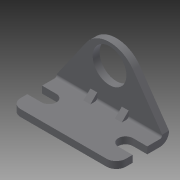
# Autodesk Inventor part: D-770
Saved by Autodesk Inventor 2013 (Build 170138000, 138)
## iProperties
Category: PARTsolutions
Company: BIMBA
Created: 2013-01-26
Part Number: D-770
Material: Generic
Catalog Web Link: www.cadenas.de
Description: Mounting Brackets for Original Line Cylinders-
Vendor: BIMBA
Document SubType Name: Modeling
Designer: actoennies
Manufacturer: BIMBA
Density: 1 g/cm^3
Mass: 1.92593 g
Surface Area: 20.9427 cm^2
Volume: 1.92593 cm^3
PSOL_IDENT_0: {\\10.0.0.242\data_v9\23d-libs\bimba\bimba\bimba_imperial\bimba_full_line\original_line_cylinders\ac
PSOL_IDENT_1: cessories\mounting_bracket.prj},191 {VTYP=3D},{NB=D-770},{LINA=D-770},{NN=Mounting Brackets for Orig
PSOL_IDENT_2: inal Line Cylinders},{DATE=26.09.2012 12:25:43},{GEOMDATE=27.08.2012 00:00:00},{VERSION=},{LINEID=40
PSOL_IDENT_3: },{LINESUBID=-1},{WBVAR=}  {NB=D-770},{LINA=D-770},{KT=DUMMY},{PN=D-770},{PSPN=0.44 (D-770)},{PN1=D-
PSOL_IDENT_4: 770},{MAT=Zinc-Plated Carbon Steel},{A=0.83},{A1=0.82900},{B=1.38},{B1=1.37500},{C=0.69},{C1=0.69000
PSOL_IDENT_5: },{D=0.44},{D1=0.44050},{E=0.19},{E1=0.19200},{F=0.38},{F1=0.38000},{G=0.56},{G1=0.56170},{H=0.09},{
PSOL_IDENT_6: H1=0.08970},{I=0.38},{I1=0.37500},{J=1.00},{J1=1.00000},{K=0.13},{K1=0.12500},{L=0.13},{L1=0.12500},
PSOL_IDENT_7: {M=0.03100},{N=0.00000},{SHP=3},{ASSCFGPRA=mounting_bracket3},{COLOR=0.75,0.75,0.75,0.00}
CNS_NB: D-770
CNS_NBSYN: $PN1.
CNS_LINA: D-770
CNS_PN: D-770
CNS_PSPN: ø.44 (D-770)
CNS_PN1: D-770
CNS_MAT: Zinc-Plated Carbon Steel
CNS_A: 0.83
CNS_A1: 0.82900
CNS_B: 1.38
CNS_B1: 1.37500
CNS_C: 0.69
CNS_C1: 0.69000
CNS_D: 0.44
CNS_D1: 0.44050
CNS_E: 0.19
CNS_E1: 0.19200
CNS_F: 0.38
CNS_F1: 0.38000
CNS_G: 0.56
CNS_G1: 0.56170
CNS_H: 0.09
CNS_H1: 0.08970
CNS_I: 0.38
CNS_I1: 0.37500
CNS_J: 1.00
CNS_J1: 1.00000
CNS_K: 0.13
CNS_K1: 0.12500
CNS_L: 0.13
CNS_L1: 0.12500
CNS_M: 0.03100
CNS_N: 0.00000
CNS_SHP: 3
CNS_ASSCFGPRA: mounting_bracket3
CNS_COLOR: 0.75,0.75,0.75,0.00
SUPPLIER: BIMBA
ARTICLENO: D-770
BOMINFO: D-770
CREATOR: CADENAS GmbH
Title: D-770
Author: Cadenas PARTsolutions
Autodesk Inventor part; units mm, degrees
sketch "Sketch_1" plane through (0, 0, 0) normal (1, 0, 0) x (0, 1, 0)
  line L0 (0, 17.526) -> (0, 3.0658)
  arc A0 (0, 3.0658) -> (3.0658, 0) centre (3.0658, 3.0658) ccw
  line L1 (3.0658, 0) -> (25.2679, 0)
  line L2 (25.2679, 0) -> (25.2679, 2.2784)
  line L3 (25.2679, 2.2784) -> (3.0658, 2.2784)
  arc A1 (2.2784, 3.0658) -> (3.0658, 2.2784) centre (3.0658, 3.0658) ccw
  line L4 (2.2784, 3.0658) -> (2.2784, 17.526)
  line L5 (2.2784, 17.526) -> (0, 17.526)
  constraints: 12 end point, 4 point on circle, 2 centre point
extrude "Extrusion1" add sketch "Sketch_1" along normal blind 34.925
sketch "Sketch_2" plane through (0, 0, 0) normal (0, 0, 1) x (1, 0, 0)
  line L0 (-6.985, -2.1057) -> (41.91, -2.1057)
  line L1 (41.91, -2.1057) -> (41.91, 33.6906)
  line L2 (41.91, 33.6906) -> (-6.985, 33.6906)
  line L3 (-6.985, 33.6906) -> (-6.985, -2.1057)
  line L4 (-2.2193, 0) -> (37.1443, 0)
  line L5 (37.1443, 0) -> (25.2694, 16.9886)
  arc A0 (25.2694, 16.9886) -> (9.6556, 16.9886) centre (17.4625, 11.5316) ccw
  line L6 (9.6556, 16.9886) -> (-2.2193, 0)
  constraints: 14 end point, 2 point on circle, 1 centre point
extrude "Extrusion2" cut sketch "Sketch_2" along normal blind 3.4176
sketch "Sketch3" plane through (34.925, 3.0658, 0) normal (0, 0, -1) x (-1, 0, 0)
  point P0 (17.4625, 11.2014)
hole "Drilling 1" at (17.4625, 14.2672, 0) direction (0, 0, 1) diameter 11.1887 depth 3.4176
sketch "Sketch_6" plane through (0, 0, 0) normal (0, 1, 0) x (-1, 0, 0)
  line L0 (17.4625, 14.351) -> (17.4625, 22.352)
  line L1 (17.4625, 22.352) -> (-3.175, 22.352)
  line L2 (-3.175, 22.352) -> (-3.175, 17.526)
  arc A0 (0, 14.351) -> (-3.175, 17.526) centre (-3.175, 14.351) ccw
  line L3 (0, 14.351) -> (17.4625, 14.351)
  constraints: 8 end point, 2 point on circle, 1 centre point
extrude "Extrusion3" cut sketch "Sketch_6" along normal blind 3.4176
sketch "Sketch_7" plane through (0, 0, 0) normal (0, 1, 0) x (-1, 0, 0)
  line L0 (-31.75, 22.352) -> (-52.3875, 22.352)
  line L1 (-52.3875, 22.352) -> (-52.3875, 14.351)
  line L2 (-52.3875, 14.351) -> (-34.925, 14.351)
  arc A0 (-31.75, 17.526) -> (-34.925, 14.351) centre (-31.75, 14.351) ccw
  line L3 (-31.75, 17.526) -> (-31.75, 22.352)
  constraints: 8 end point, 2 point on circle, 1 centre point
extrude "Extrusion4" cut sketch "Sketch_7" along normal blind 3.4176
sketch "Sketch_8" plane through (0, 0, 0) normal (0, 1, 0) x (-1, 0, 0)
  line L0 (3.4925, 12.0904) -> (-4.7625, 12.0904)
  arc A0 (-4.7625, 12.0904) -> (-4.7625, 7.2136) centre (-4.7625, 9.652) ccw
  line L1 (-4.7625, 7.2136) -> (3.4925, 7.2136)
  line L2 (3.4925, 7.2136) -> (3.4925, 12.0904)
  constraints: 6 end point, 2 point on circle, 1 centre point
extrude "Extrusion5" cut sketch "Sketch_8" along normal blind 3.4176
sketch "Sketch_9" plane through (0, 0, 0) normal (0, 1, 0) x (-1, 0, 0)
  arc A0 (-30.1625, 7.2136) -> (-30.1625, 12.0904) centre (-30.1625, 9.652) ccw
  line L0 (-30.1625, 12.0904) -> (-38.4175, 12.0904)
  line L1 (-38.4175, 12.0904) -> (-38.4175, 7.2136)
  line L2 (-38.4175, 7.2136) -> (-30.1625, 7.2136)
  constraints: 6 end point, 2 point on circle, 1 centre point
extrude "Extrusion6" cut sketch "Sketch_9" along normal blind 3.4176
sketch "Sketch_10" plane through (11.1125, 0, 0) normal (1, 0, 0) x (0, 0, -1)
  arc A0 (-4.5568, 1.8456) -> (-1.8456, 4.5568) centre (-3.0658, 3.0658) ccw
  line L0 (-1.8456, 4.5568) -> (-2.2784, 4.5568)
  line L1 (-2.2784, 4.5568) -> (-4.5568, 2.2784)
  line L2 (-4.5568, 2.2784) -> (-4.5568, 1.8456)
  constraints: 6 end point, 2 point on circle, 1 centre point
extrude "Extrusion7" add sketch "Sketch_10" along normal blind 2.2784
sketch "Sketch_14" plane through (23.8125, 0, 0) normal (1, 0, 0) x (0, 0, -1)
  arc A0 (-4.5568, 1.8456) -> (-1.8456, 4.5568) centre (-3.0658, 3.0658) ccw
  line L0 (-1.8456, 4.5568) -> (-2.2784, 4.5568)
  line L1 (-2.2784, 4.5568) -> (-4.5568, 2.2784)
  line L2 (-4.5568, 2.2784) -> (-4.5568, 1.8456)
  constraints: 6 end point, 2 point on circle, 1 centre point
extrude "Extrusion8" add sketch "Sketch_14" against normal blind 2.2784
ref_plane "h1_XY" through (17.4625, 0, 17.526) normal (1, 0, 0) x (0, 0, -1)
ref_plane "h1_YZ" through (17.4625, 0, 17.526) normal (0, 0, -1) x (0, 1, 0)
ref_plane "h1_ZX" through (17.4625, 0, 17.526) normal (0, 1, 0) x (1, 0, 0)
ref_plane "d1_XY" through (17.4625, 8.6728, 0) normal (1, 0, 0) x (0, 0, -1)
ref_plane "d1_YZ" through (17.4625, 8.6728, 0) normal (0, 0, -1) x (0, 1, 0)
ref_plane "d1_ZX" through (17.4625, 8.6728, 0) normal (0, 1, 0) x (1, 0, 0)
ref_plane "h2_XY" through (17.4625, 2.2784, 17.526) normal (1, 0, 0) x (0, 0, -1)
ref_plane "h2_YZ" through (17.4625, 2.2784, 17.526) normal (0, 0, -1) x (0, 1, 0)
ref_plane "h2_ZX" through (17.4625, 2.2784, 17.526) normal (0, 1, 0) x (1, 0, 0)
ref_plane "d2_XY" through (17.4625, 19.8615, 0) normal (1, 0, 0) x (0, 0, -1)
ref_plane "d2_YZ" through (17.4625, 19.8615, 0) normal (0, 0, -1) x (0, 1, 0)
ref_plane "d2_ZX" through (17.4625, 19.8615, 0) normal (0, 1, 0) x (1, 0, 0)
ref_plane "h3_XY" through (17.4625, 14.2672, 2.2784) normal (1, 0, 0) x (0, 0, -1)
ref_plane "h3_YZ" through (17.4625, 14.2672, 2.2784) normal (0, 0, -1) x (0, 1, 0)
ref_plane "h3_ZX" through (17.4625, 14.2672, 2.2784) normal (0, 1, 0) x (1, 0, 0)
ref_plane "h4_XY" through (17.4625, 21.0566, 2.2784) normal (1, 0, 0) x (0, 0, -1)
ref_plane "h4_YZ" through (17.4625, 21.0566, 2.2784) normal (0, 0, -1) x (0, 1, 0)
ref_plane "h4_ZX" through (17.4625, 21.0566, 2.2784) normal (0, 1, 0) x (1, 0, 0)
ref_plane "h5_XY" through (34.925, 3.175, 0) normal (1, 0, 0) x (0, 0, -1)
ref_plane "h5_YZ" through (34.925, 3.175, 0) normal (0, 0, -1) x (0, 1, 0)
ref_plane "h5_ZX" through (34.925, 3.175, 0) normal (0, 1, 0) x (1, 0, 0)
ref_plane "h6_XY" through (34.925, 0, 0) normal (1, 0, 0) x (0, 0, -1)
ref_plane "h6_YZ" through (34.925, 0, 0) normal (0, 0, -1) x (0, 1, 0)
ref_plane "h6_ZX" through (34.925, 0, 0) normal (0, 1, 0) x (1, 0, 0)
ref_plane "l1_XY" through (0, 0, 0) normal (0, 1, 0) x (1, 0, 0)
ref_plane "l1_YZ" through (0, 0, 0) normal (1, 0, 0) x (0, 0, -1)
ref_plane "l1_ZX" through (0, 0, 0) normal (0, 0, -1) x (0, 1, 0)
ref_plane "l2_XY" through (34.925, 0, 0) normal (0, 1, 0) x (1, 0, 0)
ref_plane "l2_YZ" through (34.925, 0, 0) normal (1, 0, 0) x (0, 0, -1)
ref_plane "l2_ZX" through (34.925, 0, 0) normal (0, 0, -1) x (0, 1, 0)
ref_plane "l3_XY" through (0, 0, 17.526) normal (0, 1, 0) x (1, 0, 0)
ref_plane "l3_YZ" through (0, 0, 17.526) normal (1, 0, 0) x (0, 0, -1)
ref_plane "l3_ZX" through (0, 0, 17.526) normal (0, 0, -1) x (0, 1, 0)
ref_plane "l4_XY" through (0, 0, 9.652) normal (0, 1, 0) x (1, 0, 0)
ref_plane "l4_YZ" through (0, 0, 9.652) normal (1, 0, 0) x (0, 0, -1)
ref_plane "l4_ZX" through (0, 0, 9.652) normal (0, 0, -1) x (0, 1, 0)
ref_plane "l5_XY" through (4.7625, 0, 9.652) normal (0, 1, 0) x (1, 0, 0)
ref_plane "l5_YZ" through (4.7625, 0, 9.652) normal (1, 0, 0) x (0, 0, -1)
ref_plane "l5_ZX" through (4.7625, 0, 9.652) normal (0, 0, -1) x (0, 1, 0)
ref_plane "l6_XY" through (30.1625, 0, 9.652) normal (0, 1, 0) x (1, 0, 0)
ref_plane "l6_YZ" through (30.1625, 0, 9.652) normal (1, 0, 0) x (0, 0, -1)
ref_plane "l6_ZX" through (30.1625, 0, 9.652) normal (0, 0, -1) x (0, 1, 0)
ref_plane "l7_XY" through (30.1625, 0, 12.0904) normal (0, 1, 0) x (1, 0, 0)
ref_plane "l7_YZ" through (30.1625, 0, 12.0904) normal (1, 0, 0) x (0, 0, -1)
ref_plane "l7_ZX" through (30.1625, 0, 12.0904) normal (0, 0, -1) x (0, 1, 0)
ref_plane "l8_XY" through (30.1625, 0, 7.2136) normal (0, 1, 0) x (1, 0, 0)
ref_plane "l8_YZ" through (30.1625, 0, 7.2136) normal (1, 0, 0) x (0, 0, -1)
ref_plane "l8_ZX" through (30.1625, 0, 7.2136) normal (0, 0, -1) x (0, 1, 0)
ref_plane "mounting_bracket_XY" through (17.4625, 14.2672, 2.2784) normal (0, 0, 1) x (1, 0, 0)
ref_plane "mounting_bracket_YZ" through (17.4625, 14.2672, 2.2784) normal (1, 0, 0) x (0, 1, 0)
ref_plane "mounting_bracket_ZX" through (17.4625, 14.2672, 2.2784) normal (0, 1, 0) x (0, 0, 1)
ref_plane "mounting_bracket_1_XY" through (17.4625, 14.2672, 0) normal (0, 0, 1) x (1, 0, 0)
ref_plane "mounting_bracket_1_YZ" through (17.4625, 14.2672, 0) normal (1, 0, 0) x (0, 1, 0)
ref_plane "mounting_bracket_1_ZX" through (17.4625, 14.2672, 0) normal (0, 1, 0) x (0, 0, 1)
body "Solid1"
